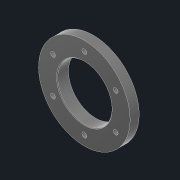
# Autodesk Inventor part: scara-base1
Saved by Autodesk Inventor 2022 (Build 260153000, 153)
## iProperties
Created: 2021-07-25
Part Number: scara-base1
Material: ABS プラスチック
Document SubType Name: Modeling
Designer: yuto6
Density: 1.06 g/cm^3
Appearance: 滑らか - 黒
Mass: 58.6832 g
Surface Area: 155.666 cm^2
Volume: 55.3615 cm^3
Description: 印刷
購入先: 印刷
在庫数: 0.0
Author: yuto6
Autodesk Inventor part; units mm, degrees
ref_plane "YZ Plane" through (0, 0, 0) normal (1, 0, 0) x (0, 1, 0)
ref_plane "XZ Plane" through (0, 0, 0) normal (0, 1, 0) x (-1, 0, 0)
ref_plane "XY Plane" through (0, 0, 0) normal (0, 0, 1) x (1, 0, 0)
sketch "スケッチ2" plane through (0, 0, 0) normal (1, 0, 0) x (0, 1, 0)
  line L0 (24.1, 0) -> (24.1, -10)
  line L1 (40.5, 0) -> (40.5, -8)
  line L2 (40.5, 0) -> (24.1, 0)
  line L3 (24.1, 0) -> (59, 0)
  line L4 (24.1, -10) -> (27, -10)
  line L5 (0, -12) -> (0, 2) projected
  line L6 (27, -10) -> (27, -8)
  line L7 (27, -8) -> (40.5, -8)
  point P0 (0, 0)
  dimension "d40" = 24.1
  dimension "d41" = 8
  dimension "d42" = 40.5
  dimension "d43" = 27
  dimension "d44" = 2
  constraints: 14 end point, 3 horizontal, 3 perpendicular, 1 horizontal alignment, 1 vertical
  measures "d40" distance from line of point (0, 0) L0
  measures "d41" distance of L1.end L1.start
  measures "d42" distance from line of point (0, 0) L1
  measures "d43" distance between parallel lines of L5 L6
  measures "d44" distance of L4.end L6.end
revolve "回転1" add sketch "スケッチ2" angle 360 about axis through (0, 0, -10) along (0, 0, 1)
sketch "スケッチ4" plane through (0, 0, 0) normal (0, 0, 1) x (1, 0, 0)
  point P0 (0, 0)
  point P1 (0, 32)
  point P2 (-27.7128, 16)
  point P3 (-27.7128, -16)
  point P4 (0, -32)
  point P5 (27.7128, -16)
  point P6 (27.7128, 16)
  dimension "d11" = 32
  dimension "d14" = 360
  constraints: 7 other
  measures "d11" distance of point (0, 0) point (0, 32)
hole "穴1" at (0, 32, 0) at (-27.7128, 16, 0) at (-27.7128, -16, 0) at (0, -32, 0) at (27.7128, -16, 0) at (27.7128, 16, 0) direction (0, 0, -1) diameter 4.3 end through all clearance for "Socket Head Cap Screw" size "M4" standard "Ansi Metric M Profile"
chamfer "面取り3" distance 0.5 angle 45 1 edges at (0, -27, -10)
chamfer "面取り4" distance 0.5 angle 45 1 edges at (0, -24.1, 0)
sketch "スケッチ9" plane through (0, 0, -8) normal (0, 0, -1) x (-1, 0, 0)
  circle A0 centre (0, -32) radius 2.15 projected
  circle A1 centre (0, 32) radius 2.15 projected
  circle A2 centre (0, -32) radius 2.15 projected
  circle A3 centre (0, -32) radius 4
  circle A4 centre (0, 32) radius 4
  point P0 (0, 0)
  dimension "d64" = 8
  dimension "d65" = 8
  constraints: 2 centre point, 2 coincident
  measures "d64" diameter of A3
  measures "d65" diameter of A4
extrude "押し出し5" cut sketch "スケッチ9" against normal blind 4.2 contours A0 | A1 | A3 | A4
